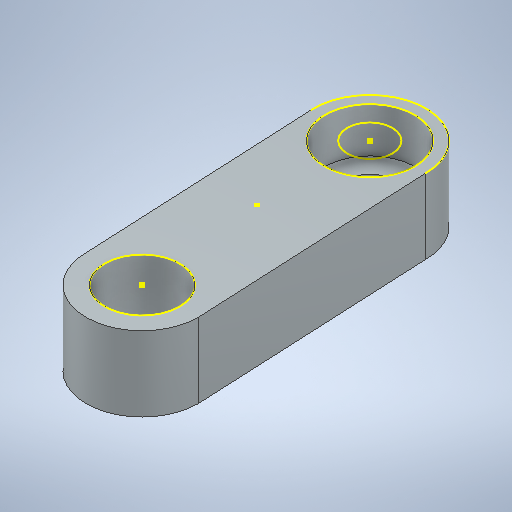
# Autodesk Inventor part: Redesign_Linkage
Saved by Autodesk Inventor 2025.2 (Build 292293000, 293)
## iProperties
Created: 2024-12-26
Part Number: Redesign_Linkage
Material: Generic
Document SubType Name: Modeling
Designer: m_kni
Density: 1 g/cm^3
Appearance: Default
Author: m_kni
## iProperties of the stored document Redesign_Linkage_3DPrint.ipt
Created: 2025-01-30
Part Number: Redesign_Linkage_3DPrint
Material: Generic
Document SubType Name: Modeling
Designer: m_kni
Density: 1 g/cm^3
Appearance: Default
Author: m_kni
Autodesk Inventor part; units mm, degrees
ref_plane "YZ Plane" through (0, 0, 0) normal (1, 0, 0) x (0, 1, 0)
ref_plane "XZ Plane" through (0, 0, 0) normal (0, 1, 0) x (-1, 0, 0)
ref_plane "XY Plane" through (0, 0, 0) normal (0, 0, 1) x (1, 0, 0)
sketch "Sketch1" plane through (0, 0, 0) normal (0, 1, 0) x (-1, 0, 0)
  circle A0 centre (-0.749959, 8.455141) radius 2.5
  circle A1 centre (0, -7.527273) radius 1.5
  circle A2 centre (-0.749959, 8.455141) radius 3.75
  circle A3 centre (0, -7.527273) radius 3
  line L0 (3, 8.472727) -> (3, -7.527273)
  line L1 (-4.499959, 8.455141) -> (-2.987099, -7.805192)
  circle A4 centre (0, -7.527273) radius 3.75
  line L2 (-4.499959, 8.455141) -> (-3.75, -7.527273)
  line L3 (3, 8.472727) -> (3.745841, -7.350712)
  point P0 (0, 0)
  dimension "d0" = 16
  dimension "d1" = 5
  dimension "d2" = 3
  dimension "d3" = 7.5
  dimension "d4" = 6
  dimension "d10" = 7.5
  constraints: 8 end point, 6 point on circle, 5 centre point, 5 coincident, 2 tangent, 1 vertical
  measures "d0" distance of point (0, -7.527) point (-0.75, 8.455)
  measures "d1" diameter of A0
  measures "d2" diameter of A1
  measures "d3" diameter of A2
  measures "d4" diameter of A3
  measures "d10" diameter of A4
sketch "Sketch1 outline for Extrusion1" plane through (0, 0, 0) normal (0, 1, 0) x (-1, 0, 0)
  arc A0 (3, 8.472727) -> (-4.499959, 8.455141) centre (-0.749959, 8.455141) ccw
  line L0 (-4.499959, 8.455141) -> (-3.75, -7.527273)
  arc A1 (-3.75, -7.527273) -> (3.745841, -7.350712) centre (0, -7.527273) ccw
  line L1 (3.745841, -7.350712) -> (3, 8.472727)
  circle A2 centre (0, -7.527273) radius 1.5
  circle A3 centre (-0.749959, 8.455141) radius 2.5
extrude "Extrusion1" add sketch "Sketch1 outline for Extrusion1" along normal blind 5
sketch "Sketch2" plane through (0, 5, 0) normal (0, 1, 0) x (1, 0, 0)
  circle A0 centre (0, 7.527273) radius 1.5
  circle A1 centre (0, 7.527273) radius 3
  point P0 (0, 0)
  point P1 (3, 7.527273)
  dimension "d7" = 6
  constraints: 1 centre point, 1 coincident
  measures "d7" diameter of A1
extrude "Extrusion2" cut sketch "Sketch2" against normal blind 3
sketch "Sketch3" plane through (0, 5, 0) normal (0, 1, 0) x (1, 0, 0)
  circle A0 centre (0.749959, -8.455141) radius 2.5
  circle A1 centre (0, 7.527273) radius 3
  circle A2 centre (0, 7.527273) radius 1.5
  arc A3 (3.75, 7.527273) -> (-3.745841, 7.350712) centre (0, 7.527273) ccw
  point P0 (0, 0)
body "Solid1"
